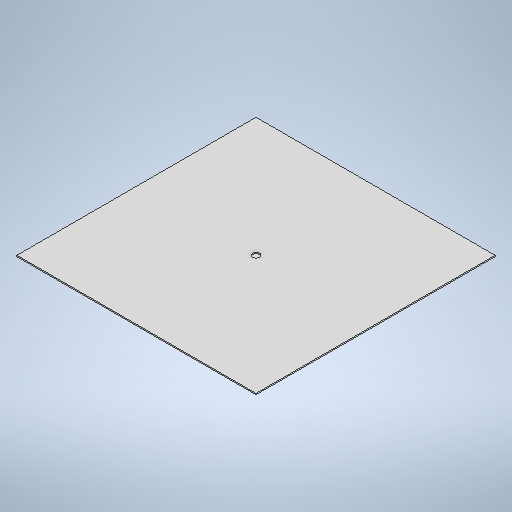
# Autodesk Inventor part: StatorGroundPlate
Saved by Autodesk Inventor 2025.1 (Build 291241000, 241)
## iProperties
Created: 2025-10-21
Part Number: StatorGroundPlate
Material: Generic
Document SubType Name: Modeling
Designer: jonas
Density: 1 g/cm^3
Appearance: Default
Author: jonas
Autodesk Inventor part; units mm, degrees
ref_plane "YZ Plane" through (0, 0, 0) normal (1, 0, 0) x (0, 1, 0)
ref_plane "XZ Plane" through (0, 0, 0) normal (0, 1, 0) x (-1, 0, 0)
ref_plane "XY Plane" through (0, 0, 0) normal (0, 0, 1) x (1, 0, 0)
sketch "Sketch1" plane through (0, 0, 0) normal (0, 1, 0) x (-1, 0, 0)
  circle A0 centre (0, 0) radius 438.1 construction
  line L0 (500, -500) -> (-500, -500)
  line L1 (-500, -500) -> (-500, 500)
  line L2 (-500, 500) -> (500, 500)
  line L3 (500, 500) -> (500, -500)
  line L4 (0, -248.7708) -> (0, 248.7708) construction
  line L5 (-1768.3221, 0) -> (1768.3221, 0) construction
  circle A1 centre (0, 0) radius 15
  dimension "d0" = 876.2
  dimension "d1" = 1000
  dimension "d2" = 1000
  dimension "d5" = 30
  constraints: 12 end point, 3 coincident, 2 centre point, 2 horizontal, 2 midpoint, 2 parallel, 1 perpendicular, 1 vertical, 2 other
  measures "d0" diameter of A0
  measures "d1" distance of L2.end L0.start
  measures "d2" distance of L0.start L0.end
  measures "d5" diameter of A1
extrude "Extrusion1" add sketch "Sketch1" along normal blind 5
body "Solid1"
